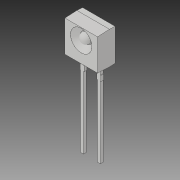
# Autodesk Inventor part: IR Emitter TSKS5400S
Saved by Autodesk Inventor 2017.3 (Build 213256000, 256)
## iProperties
Part Number: IR Emitter TSKS5400S
Material: Generisch
Document SubType Name: Modeling
Designer: rYan
Density: 1 g/cm^3
Appearance: Vorgabe
Author: rYan
Autodesk Inventor part; units mm, degrees
ref_plane "YZ Plane" through (0, 0, 0) normal (1, 0, 0) x (0, 1, 0)
ref_plane "XZ Plane" through (0, 0, 0) normal (0, 1, 0) x (-1, 0, 0)
ref_plane "XY Plane" through (0, 0, 0) normal (0, 0, 1) x (1, 0, 0)
sketch "Skizze1" plane through (0, 0, 0) normal (1, 0, 0) x (0, 1, 0)
  line L0 (0.85, 1.755453) -> (0, 1.8)
  line L1 (0, 1.8) -> (-1.8, 1.705666)
  line L2 (-1.8, 1.705666) -> (-1.8, -3.005666)
  line L3 (-1.8, -3.005666) -> (0, -3.1)
  line L4 (0, -3.1) -> (0.85, -3.055453)
  line L5 (0.85, -3.055453) -> (0.85, 1.755453)
  line L6 (0, 2.78) -> (0, -4.08)
  line L7 (-2.33, 0) -> (1.38, 0)
  point P0 (0, 0)
  dimension "d0" = 2.65
  dimension "d1" = 4.9
  dimension "d2" = 3.1
  dimension "d3" = 3
  dimension "d4" = 3
  dimension "d5" = 3
  dimension "d6" = 3
  dimension "d7" = 1.8
  constraints: 12 end point, 2 point on line, 1 parallel, 1 vertical
  measures "d0" distance between parallel lines of L2 L5
  measures "d1" distance of L3.end L0.end
  measures "d2" distance from line of L3.end L7
  measures "d3" angle of L7 L1
  measures "d4" angle of L0 L7
  measures "d5" angle of L4 L7
  measures "d6" angle of L7 L3
  measures "d7" distance between parallel lines of L6 L2
sketch "Skizze1 outline for Extrusion1" plane through (0, 0, 0) normal (1, 0, 0) x (0, 1, 0)
  line L0 (0.85, 1.755453) -> (0, 1.8)
  line L1 (0, 1.8) -> (-1.8, 1.705666)
  line L2 (-1.8, 1.705666) -> (-1.8, -3.005666)
  line L3 (-1.8, -3.005666) -> (0, -3.1)
  line L4 (0, -3.1) -> (0.85, -3.055453)
  line L5 (0.85, -3.055453) -> (0.85, 1.755453)
extrude "Extrusion1" add sketch "Skizze1 outline for Extrusion1" along normal mid plane 4.9
sketch "Skizze2" plane through (0, 0, 0) normal (0, 1, 0) x (-1, 0, 0)
  line L0 (2.45, -3.1) -> (-2.45, -3.1)
  line L1 (1.495, -2.1) -> (1.045, -2.1)
  line L2 (1.045, -16) -> (1.495, -16)
  line L3 (0.97, -4.45) -> (0.97, -5.25)
  line L4 (1.57, -5.25) -> (1.57, -4.45)
  line L5 (1.57, -4.45) -> (1.495, -4.45)
  line L6 (1.045, -4.45) -> (0.97, -4.45)
  line L7 (1.495, -16) -> (1.495, -5.25)
  line L8 (1.495, -4.45) -> (1.495, -2.1)
  line L9 (1.045, -2.1) -> (1.045, -4.45)
  line L10 (1.045, -5.25) -> (1.045, -16)
  line L11 (0.97, -5.25) -> (1.045, -5.25)
  line L12 (1.495, -5.25) -> (1.57, -5.25)
  line L13 (1.27, -16) -> (1.27, -2.1) construction
  line L14 (2.45, 1.8) -> (-2.45, 1.8) construction
  line L15 (-2.45, 1.755453) -> (-2.45, 1.8) construction
  line L16 (2.45, 1.755453) -> (-2.45, 1.755453) construction
  line L17 (2.45, 1.8) -> (2.45, 1.755453) construction
  point P0 (0, 0)
  dimension "d10" = 0.45
  dimension "d11" = 0.6
  dimension "d12" = 0.8
  dimension "d13" = 2.15
  dimension "d14" = 1.27
  dimension "d15" = 17.8
  dimension "d16" = 1
  constraints: 26 end point, 10 parallel, 4 perpendicular, 3 horizontal, 2 collinear, 2 midpoint, 3 other
  measures "d10" distance between parallel lines of L8 L9
  measures "d11" distance between parallel lines of L3 L4
  measures "d12" distance of L3.start L3.end
  measures "d13" distance between parallel lines of L11 L0
  measures "d14" distance from line of point (0, 0) L13
  measures "d15" distance between parallel lines of L2 L14
  measures "d16" distance between parallel lines of L1 L0
sketch "Skizze2 outline for Extrusion2" plane through (0, 0, 0) normal (0, 1, 0) x (-1, 0, 0)
  line L0 (1.495, -4.45) -> (1.495, -2.1)
  line L1 (1.57, -4.45) -> (1.495, -4.45)
  line L2 (1.57, -5.25) -> (1.57, -4.45)
  line L3 (1.495, -5.25) -> (1.57, -5.25)
  line L4 (1.495, -16) -> (1.495, -5.25)
  line L5 (1.045, -16) -> (1.495, -16)
  line L6 (1.045, -5.25) -> (1.045, -16)
  line L7 (0.97, -5.25) -> (1.045, -5.25)
  line L8 (0.97, -4.45) -> (0.97, -5.25)
  line L9 (1.045, -4.45) -> (0.97, -4.45)
  line L10 (1.045, -2.1) -> (1.045, -4.45)
  line L11 (1.495, -2.1) -> (1.045, -2.1)
extrude "Extrusion2" add sketch "Skizze2 outline for Extrusion2" against normal blind 0.4
mirror "Spiegeln1" about plane through (0, 0, 0) normal (1, 0, 0) of "Extrusion2"
sketch "Skizze3" plane through (-2.45, -1.8, -3.005666) normal (0, -1, 0) x (1, 0, 0)
  line L0 (2.45, 5.785666) -> (2.45, -1.074334)
  line L1 (-0.98, 3.005666) -> (5.88, 3.005666)
  circle A0 centre (2.45, 3.005666) radius 1.6
  dimension "d19" = 3.2
  constraints: 1 centre point, 1 coincident
  measures "d19" diameter of A0
sketch "Skizze3 outline for Extrusion3" plane through (-2.45, -1.8, -3.005666) normal (0, -1, 0) x (1, 0, 0)
  circle A0 centre (2.45, 3.005666) radius 1.6
extrude "Extrusion3" cut sketch "Skizze3 outline for Extrusion3" against normal blind 0.75 draft -45
sketch "Skizze4" plane through (0, 0, 0) normal (1, 0, 0) x (0, 1, 0)
  line L0 (-1.05, 0.85) -> (-1.05, -0.85)
  arc A0 (-1.05, 0.75) -> (-1.05, -0.75) centre (-1.05, 0) ccw
  line L1 (-2.371105, 0) -> (1.386851, 0)
  line L2 (-1.05, 0.75) -> (-1.05, -0.75)
  point P0 (0, 0)
  dimension "d22" = 0.75
  constraints: 3 point on line, 2 end point, 2 point on circle, 1 centre point, 1 collinear, 1 midpoint
  measures "d22" radius of A0
sketch "Skizze4 outline for Umdrehung1" plane through (0, 0, 0) normal (1, 0, 0) x (0, 1, 0)
  line L0 (-1.05, -0.75) -> (-1.05, 0.75)
  arc A0 (-1.05, 0.75) -> (-1.05, -0.75) centre (-1.05, 0) ccw
revolve "Umdrehung1" add sketch "Skizze4 outline for Umdrehung1" angle 180 mid plane about axis through (0, -1.05, 0.75) along (0, 0, -1)
